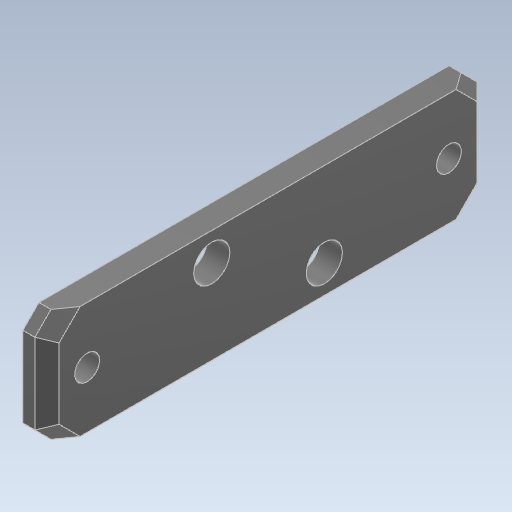
# Autodesk Inventor part: realsense_adapter
Saved by Autodesk Inventor 2024 (Build 280153000, 153)
## iProperties
Created: 2023-09-30
Part Number: realsense_adapter
Material: ABS プラスチック
Document SubType Name: Modeling
Designer: michi
Density: 1.06 g/cm^3
Appearance: 滑らか - 黒
Author: michi
Autodesk Inventor part; units mm, degrees
ref_plane "YZ Plane" through (0, 0, 0) normal (1, 0, 0) x (0, 1, 0)
ref_plane "XZ Plane" through (0, 0, 0) normal (0, 1, 0) x (-1, 0, 0)
ref_plane "XY Plane" through (0, 0, 0) normal (0, 0, 1) x (1, 0, 0)
sketch "スケッチ1" plane through (0, 0, 0) normal (1, 0, 0) x (0, 1, 0)
  line L0 (-7, 27.5) -> (7, 27.5)
  line L1 (7, 27.5) -> (7, -27.5)
  line L2 (7, -27.5) -> (-7, -27.5)
  line L3 (-7, -27.5) -> (-7, 27.5)
  line L4 (-7, 27.5) -> (7, -27.5) construction
  line L5 (7, 27.5) -> (-7, -27.5) construction
  circle A0 centre (0, 22.5) radius 1.55
  circle A1 centre (0, -22.5) radius 1.55
  circle A2 centre (3.5, 7) radius 2.25
  circle A3 centre (-3.5, -7) radius 2.25
  line L6 (-7, -14) -> (7, 14) construction
  line L7 (0.253, -0.1265) -> (-0.253, 0.1265) construction
  line L8 (0, 27.5) -> (0, -27.5) construction
  line L9 (7, 0) -> (-7, 0) construction
  circle A4 centre (3.5, 7) radius 3
  circle A5 centre (-3.5, -7) radius 3
  line L10 (-7, -10) -> (7, -10) construction
  line L11 (-7, 10) -> (7, 10) construction
  point P0 (0, 0)
  dimension "d0" = 45
  dimension "d1" = 14
  dimension "d2" = 55
  dimension "d5" = 4.5
  dimension "d6" = 3.1
  dimension "d11" = 6
  dimension "d23" = 20
  dimension "d24" = 7
  constraints: 24 end point, 10 point on line, 8 midpoint, 6 centre point, 4 parallel, 2 equal radius, 2 tangent, 1 horizontal, 1 perpendicular, 2 other
  measures "d0" distance of A1.centre A0.centre
  measures "d1" distance of L0.start L0.end
  measures "d2" distance of L0.end L1.end
  measures "d5" diameter of A2
  measures "d6" diameter of A0
  measures "d11" diameter of A4
  measures "d23" distance between parallel lines of L11 L10
  measures "d24" horizontal distance of A2.centre A3.centre
sketch "スケッチ2" plane through (0, 0, 0) normal (0, 0, 1) x (1, 0, 0)
  line L0 (0, 7) -> (3, 7)
  line L1 (3, 7) -> (3, -7)
  line L2 (3, -7) -> (0, -7)
  line L3 (0, -7) -> (0, 7)
  line L4 (0.2, 7) -> (0.2, -7) construction
  line L5 (0, -7) -> (0, 7) construction
  point P0 (0, 0)
  dimension "d7" = 2.8
  dimension "d8" = 0.2
  constraints: 10 end point, 4 point on line, 2 parallel, 1 collinear, 1 horizontal, 1 perpendicular
  measures "d7" distance between parallel lines of L1 L4
  measures "d8" distance between parallel lines of L3 L4
extrude "押し出し1" add sketch "スケッチ1" along normal up to surface (3 mm away) contours L0 L1 L2 L3 | A0 | A1 | A2 | A3 | A4 | A5
extrude "押し出し2" cut sketch "スケッチ1" along normal through all contours A0 | A1 | A2 | A3
extrude "押し出し3" cut sketch "スケッチ1" along normal up to surface (0.2 mm away) contours A2 | A3 | A4 | A5
chamfer "面取り1" distance 2 angle 45 4 edges at (1.5, 7, -27.5) (1.5, 7, 27.5) (1.5, -7, 27.5) (1.5, -7, -27.5)
chamfer "面取り2" distance 1.5 angle 45 6 edges at (3, 0, -27.5) (3, -6, -26.5) (3, -6, 26.5) (3, 0, 27.5) (3, 6, 26.5) (3, 6, -26.5)
equation "\"d6\" = d_hole_M3"
equation "\"d11\" = d_spothole_M3"
equation "\"d_hole_M5\" = 5.2"
equation "\"d_hole_M4\" = 4.1"
equation "\"d_hole_M3\" = 3.1"
equation "\"d_hole_M2_5\" = 2.6"
equation "\"d_hole_M2\" = 2.1"
equation "\"d_screwhole_M4\" = 3.3"
equation "\"d_screwhole_M3\" = 2.5"
equation "\"d_spothole_M4\" = 7.5"
equation "\"d_spothole_M3\" = 6"
equation "\"d_spothole_M2_5\" = 5"
